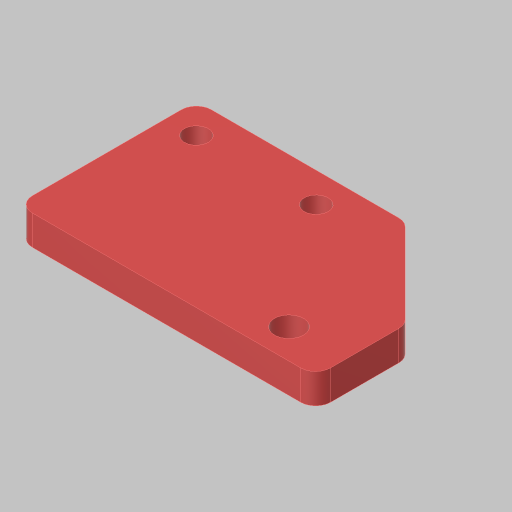
# Autodesk Inventor part: HS-002
Saved by Autodesk Inventor 2023.5 (Build 275446000, 446)
## iProperties
Created: 2025-02-22
Part Number: HS-002
Material: ABS Plastic
Document SubType Name: Modeling
Designer: slick
Density: 1.06 g/cm^3
Appearance: Smooth - Red
Author: slick
Autodesk Inventor part; units mm, degrees
ref_plane "YZ Plane" through (0, 0, 0) normal (1, 0, 0) x (0, 1, 0)
ref_plane "XZ Plane" through (0, 0, 0) normal (0, 1, 0) x (-1, 0, 0)
ref_plane "XY Plane" through (0, 0, 0) normal (0, 0, 1) x (1, 0, 0)
sketch "Sketch1" plane through (0, 0, 0) normal (0, 1, 0) x (-1, 0, 0)
  line L0 (-31.75, 19.05) -> (31.75, 19.05)
  line L1 (31.75, 19.05) -> (31.75, -19.05)
  line L2 (31.75, -19.05) -> (-31.75, -19.05)
  line L3 (-31.75, -19.05) -> (-31.75, 19.05)
  line L4 (-31.75, 19.05) -> (31.75, -19.05) construction
  line L5 (31.75, 19.05) -> (-31.75, -19.05) construction
  point P0 (0, 0)
  dimension "d0" = 63.5
  dimension "d1" = 38.1
  constraints: 12 end point, 2 midpoint, 2 parallel, 1 horizontal, 1 perpendicular
  measures "d0" distance of L1.end L2.end
  measures "d1" distance of L0.end L1.end
extrude "Extrusion1" add sketch "Sketch1" along normal blind 6.35
sketch "Sketch2" plane through (0, 6.35, 0) normal (0, 1, 0) x (1, 0, 0)
  line L0 (-25.4, 12.7) -> (0.127, 12.7) construction
  line L1 (31.75, 19.05) -> (-31.75, 19.05) construction
  line L2 (-31.75, 19.05) -> (-31.75, -19.05) construction
  point P0 (0, 0)
  point P1 (0, 12.7)
  dimension "d4" = 25.527
  dimension "d5" = 6.35
  dimension "d22" = 6.35
  constraints: 2 end point, 1 horizontal, 1 horizontal alignment, 1 vertical alignment
  measures "d4" distance of L0.start L0.end
  measures "d5" distance from line of L1 L0.start
  measures "d22" distance from line of L2 L0.start
hole "Hole1" at (-25.4, 6.35, -12.7) at (0.127, 6.35, -12.7) direction (0, -1, 0) diameter 5.1054 end through all clearance for "Flat Head Machine Screw (82)" size "#10" standard "Ansi Unified Screw Threads"
sketch "Sketch3" plane through (0, 6.35, 0) normal (0, 1, 0) x (1, 0, 0)
  line L0 (-31.75, -19.05) -> (31.75, -19.05) construction
  point P0 (0, 0)
  point P1 (19.7358, -12.7)
  dimension "d13" = 6.35
  dimension "d28" = 19.7358
  measures "d13" distance from line of L0 point (19.736, -12.7)
  measures "d28" horizontal distance of point (19.736, -12.7) point (0, 0)
hole "Hole2" at (19.7358, 6.35, 12.7) direction (0, -1, 0) diameter 6.1976 end through all
fillet "Fillet1" radius 3.175 4 edges at (-31.75, 3.175, -19.05) (31.75, 3.175, -19.05) (31.75, 3.175, 19.05) (-31.75, 3.175, 19.05)
sketch "Sketch4" plane through (0, 6.35, 0) normal (0, 1, 0) x (1, 0, 0)
  arc A0 (-31.75, -15.875) -> (-28.575, -19.05) centre (-28.575, -15.875) ccw construction
  line L0 (-31.75, -15.875) -> (-31.75, 15.875) construction
  arc A1 (-28.575, 19.05) -> (-31.75, 15.875) centre (-28.575, 15.875) ccw construction
  line L1 (-28.575, 19.05) -> (28.575, 19.05) construction
  arc A2 (31.75, 15.875) -> (28.575, 19.05) centre (28.575, 15.875) ccw construction
  line L2 (31.75, 15.875) -> (31.75, -15.875) construction
  arc A3 (28.575, -19.05) -> (31.75, -15.875) centre (28.575, -15.875) ccw construction
  line L3 (28.575, -19.05) -> (-28.575, -19.05) construction
  circle A4 centre (19.7358, -12.7) radius 3.0988 construction
  circle A5 centre (-25.4, 12.7) radius 2.5527 construction
  circle A6 centre (0.127, 12.7) radius 2.5527 construction
  line L4 (28.575, 19.05) -> (-28.575, 19.05) construction
  line L5 (12.7, 19.05) -> (31.75, 0)
  line L6 (12.7, 19.05) -> (28.575, 19.05)
  line L7 (31.75, -15.875) -> (31.75, 15.875) construction
  line L8 (31.75, 0) -> (31.75, 15.875)
  arc A7 (31.75, 15.875) -> (28.575, 19.05) centre (28.575, 15.875) ccw construction
  arc A8 (31.75, 15.875) -> (28.575, 19.05) centre (28.575, 15.875) ccw
  point P0 (0, 0)
  dimension "d23" = 19.05
  dimension "d24" = 19.05
  constraints: 6 end point, 3 point on circle, 1 centre point, 1 coincident, 1 collinear, 1 midpoint, 1 point on line
  measures "d23" distance from line of L1 L5.end
  measures "d24" distance from line of L2 L5.start
extrude "Extrusion2" cut sketch "Sketch4" against normal blind 6.35
fillet "Fillet2" radius 3.175 2 edges at (12.7, 3.175, -19.05) (31.75, 3.175, 0)
body "Solid1"
